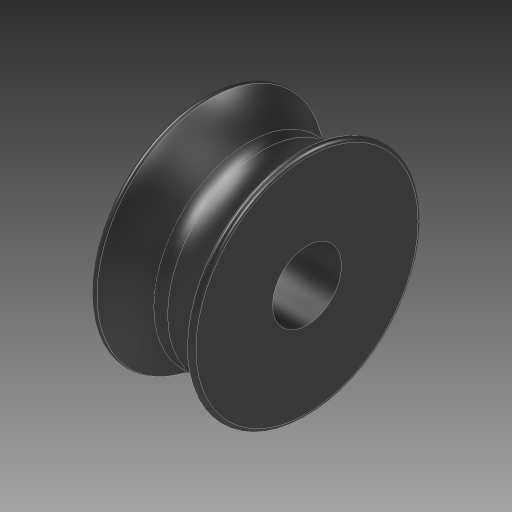
# Autodesk Inventor part: Harken 16mm V Bearing
Saved by Autodesk Inventor 2023 (Build 270158000, 158)
## iProperties
Created: 2022-05-24
Part Number: Harken 16mm V Bearing
Material: Aluminum 6061
Document SubType Name: Modeling
Designer: Cal
Density: 2.7 g/cm^3
Appearance: Glossy - Black
Author: Cal
Autodesk Inventor part; units mm, degrees
ref_plane "YZ Plane" through (0, 0, 0) normal (1, 0, 0) x (0, 1, 0)
ref_plane "XZ Plane" through (0, 0, 0) normal (0, 1, 0) x (-1, 0, 0)
ref_plane "XY Plane" through (0, 0, 0) normal (0, 0, 1) x (1, 0, 0)
sketch "Sketch1" plane through (0, 0, 0) normal (0, 0, 1) x (1, 0, 0)
  arc A0 (-0.5, 6.875) -> (0.5, 6.875) centre (0, 9.3245) ccw
  arc A1 (-3.683, 8.5929) -> (-0.5, 6.875) centre (0.75, 12.9987) ccw
  arc A2 (0.5, 6.875) -> (3.683, 8.5929) centre (-0.75, 12.9987) ccw
  line L0 (-3.683, 8.5929) -> (-3.683, 2.4892)
  line L1 (-3.683, 2.4892) -> (3.683, 2.4892)
  line L2 (3.683, 2.4892) -> (3.683, 8.5929)
  line L3 (-3.683, 0) -> (3.683, 0) construction
  point P0 (0, 0)
  point P1 (0, 0)
  dimension "d0" = 2.5
  dimension "d1" = 6.25
  dimension "d2" = 0.5
  dimension "d3" = 7.366
  dimension "d4" = 4.9784
  dimension "d5" = 13.75
  constraints: 8 end point, 6 point on circle, 3 centre point, 2 horizontal alignment, 2 perpendicular, 2 tangent, 1 coincident, 1 equal radius, 1 midpoint, 1 parallel, 1 vertical, 1 vertical alignment
  measures "d0" radius of A0
  measures "d1" radius of A1
  measures "d2" horizontal distance of A0.end A0.centre
  measures "d3" distance of L2.end L0.start
  measures "d4" diameter of L1 L3
  measures "d5" diameter of A0.start L3
revolve "Revolution1" add sketch "Sketch1" angle 360 about axis through (-3.683, 0, 0) along (1, 0, 0)
fillet "Fillet1" radius 0.254 2 edges at (-3.683, -8.5929, 0) (3.683, -8.5929, 0)
body "Solid1"
